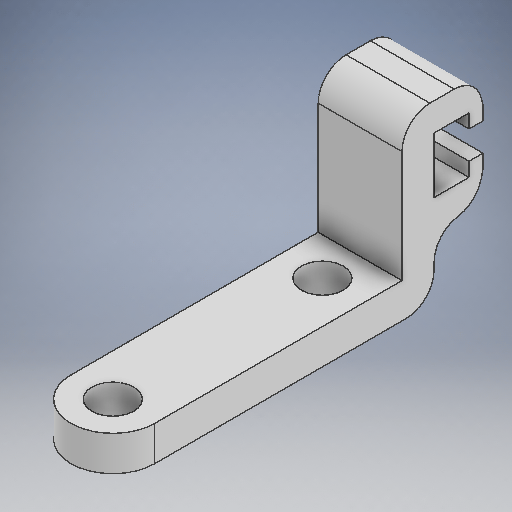
# Autodesk Inventor part: wire_holder_femur
Saved by Autodesk Inventor 2026.1 (Build 301233000, 233)
## iProperties
Created: 2025-12-05
Part Number: wire_holder_femur
Material: Generic
Document SubType Name: Modeling
Designer: emanuel
Density: 1 g/cm^3
Appearance: Default
Author: emanuel
Autodesk Inventor part; units mm, degrees
ref_plane "YZ Plane" through (0, 0, 0) normal (1, 0, 0) x (0, 1, 0)
ref_plane "XZ Plane" through (0, 0, 0) normal (0, 1, 0) x (-1, 0, 0)
ref_plane "XY Plane" through (0, 0, 0) normal (0, 0, 1) x (1, 0, 0)
sketch "Sketch1" plane through (0, 0, 0) normal (0, 1, 0) x (-1, 0, 0)
  circle A0 centre (0, 0) radius 1.5
  line L0 (0, 0) -> (0, -15)
  line L1 (0, 0) -> (15, 0) construction
  circle A1 centre (0, -15) radius 1.5
  line L2 (0, -15) -> (0, -17.5)
  line L3 (0, -17.5) -> (0, -20)
  circle A2 centre (0, 0) radius 3
  line L4 (3, 0) -> (-3, 0)
  line L5 (-3, 0) -> (-3, -20)
  line L6 (-3, -20) -> (3, -20)
  line L7 (3, -20) -> (3, 0)
  dimension "d6" = 6
  dimension "d0" = 3
  dimension "d1" = 15
  dimension "d2" = 90
  dimension "d3" = 3
  dimension "d4" = 2.5
  dimension "d5" = 2.5
  constraints: 16 end point, 3 coincident, 2 centre point, 2 horizontal, 2 parallel, 2 perpendicular, 2 point on line, 2 vertical, 3 other
  measures "d0" diameter of A0
  measures "d1" distance of L0.start L0.end
  measures "d2" angle of L0 L1
  measures "d3" diameter of A1
  measures "d4" distance of L2.start L2.end
  measures "d5" distance of L2.end L3.end
sketch "Sketch1 outline for Extrusion1" plane through (0, 0, 0) normal (0, 1, 0) x (-1, 0, 0)
  arc A0 (3, 0) -> (-3, 0) centre (0, 0) ccw
  line L0 (3, -20) -> (3, 0)
  line L1 (-3, 0) -> (-3, -20)
  line L2 (-3, -20) -> (3, -20)
  circle A1 centre (0, -15) radius 1.5
  circle A2 centre (0, 0) radius 1.5
extrude "Extrusion1" add sketch "Sketch1 outline for Extrusion1" along normal blind 2.5
sketch "Sketch2" plane through (0, 2.5, 0) normal (0, 1, 0) x (1, 0, 0)
  line L0 (3, 20) -> (-3, 20) projected
  line L1 (-3, 20) -> (3, 20)
  line L2 (3, 20) -> (3, 17.7)
  line L3 (3, 17.7) -> (-3, 17.7)
  line L4 (-3, 17.7) -> (-3, 20)
  point P0 (0, 0)
  dimension "d9" = 2.3
  constraints: 8 end point, 2 parallel, 1 horizontal, 1 perpendicular
  measures "d9" distance of L1.end L2.end
sketch "Sketch2 outline for Extrusion2" plane through (0, 2.5, 0) normal (0, 1, 0) x (1, 0, 0)
  line L0 (-3, 20) -> (-3, 17.7)
  line L1 (3, 20) -> (-3, 20)
  line L2 (3, 17.7) -> (3, 20)
  line L3 (-3, 17.7) -> (3, 17.7)
extrude "Extrusion2" add sketch "Sketch2 outline for Extrusion2" along normal blind 10
sketch "Sketch3" plane through (3, 0, -20) normal (0, 0, -1) x (-1, 0, 0)
  line L0 (0, 0) -> (0, 12.5) projected
  line L1 (6, 0) -> (6, 12.5) projected
  line L2 (0, 12.5) -> (6, 12.5)
  line L3 (6, 12.5) -> (6, 10.5)
  line L4 (6, 10.5) -> (0, 10.5)
  line L5 (0, 10.5) -> (0, 12.5)
  line L6 (0, 10.5) -> (6, 10.5)
  line L7 (6, 10.5) -> (6, 6.5)
  line L8 (6, 6.5) -> (0, 6.5)
  line L9 (0, 6.5) -> (0, 10.5)
  line L10 (0, 6.5) -> (6, 6.5)
  line L11 (6, 6.5) -> (6, 4.5)
  line L12 (6, 4.5) -> (0, 4.5)
  line L13 (0, 4.5) -> (0, 6.5)
  point P0 (3, 0)
  point P1 (0, 4.5)
  point P2 (0, 6.5)
  point P3 (0, 10.5)
  dimension "d12" = 2
  dimension "d13" = 6
  dimension "d14" = 4
  dimension "d15" = 2
  constraints: 24 end point, 6 parallel, 3 horizontal, 3 perpendicular, 2 point on line
  measures "d12" distance of L2.end L3.end
  measures "d13" distance of L7.end L8.end
  measures "d14" distance of L6.end L7.end
  measures "d15" distance of L10.end L11.end
sketch "Sketch3 outline for Extrusion3" plane through (3, 0, -20) normal (0, 0, -1) x (-1, 0, 0)
  line L0 (0, 4.5) -> (6, 4.5)
  line L1 (0, 6.5) -> (0, 4.5)
  line L2 (6, 6.5) -> (0, 6.5)
  line L3 (6, 4.5) -> (6, 6.5)
  line L4 (6, 12.5) -> (0, 12.5)
  line L5 (6, 10.5) -> (6, 12.5)
  line L6 (0, 10.5) -> (6, 10.5)
  line L7 (0, 12.5) -> (0, 10.5)
extrude "Extrusion3" add sketch "Sketch3 outline for Extrusion3" along normal blind 3
sketch "Sketch4" plane through (3, 0, 0) normal (1, 0, 0) x (0, 0, -1)
  line L0 (20, 10.5) -> (23, 10.5)
  line L1 (20, 6.5) -> (23, 6.5)
  line L2 (23, 10.5) -> (22.5, 10.5)
  line L3 (22.5, 10.5) -> (22.5, 6.5)
  line L4 (22.5, 6.5) -> (23, 6.5)
  line L5 (23, 6.5) -> (23, 10.5)
  line L6 (22.5, 10.5) -> (23.5, 10.5)
  line L7 (23.5, 10.5) -> (23.5, 9.5)
  line L8 (23.5, 9.5) -> (22.5, 9.5)
  line L9 (22.5, 9.5) -> (22.5, 10.5)
  line L10 (22.5, 6.5) -> (23.5, 6.5)
  line L11 (23.5, 6.5) -> (23.5, 7.5)
  line L12 (23.5, 7.5) -> (22.5, 7.5)
  line L13 (22.5, 7.5) -> (22.5, 6.5)
  line L14 (23, 12.5) -> (23, 10.5)
  line L15 (23.5, 10.5) -> (23, 12.5)
  line L16 (23, 12.5) -> (23, 10.5)
  line L17 (23.5, 6.5) -> (23, 4.499196)
  line L18 (23, 4.5) -> (23, 6.5)
  line L19 (23, 4.499196) -> (23, 6.5)
  point P0 (0, 0)
  dimension "d18" = 0.5
  dimension "d19" = 1
  dimension "d20" = 1
  dimension "d21" = 1
  dimension "d22" = 1
  constraints: 32 end point, 6 parallel, 3 horizontal, 3 perpendicular, 2 collinear, 1 point on line
  measures "d18" distance of L4.end L3.end
  measures "d19" distance of L7.end L8.end
  measures "d20" distance of L6.end L7.end
  measures "d21" distance of L12.end L11.end
  measures "d22" distance of L11.end L10.end
sketch "Sketch4 outline for Extrusion4" plane through (3, 0, 0) normal (1, 0, 0) x (0, 0, -1)
  line L0 (23, 4.5) -> (23.5, 6.5)
  line L1 (23, 6.5) -> (23, 4.5)
  line L2 (22.5, 6.5) -> (23, 6.5)
  line L3 (22.5, 7.5) -> (22.5, 6.5)
  line L4 (23.5, 7.5) -> (22.5, 7.5)
  line L5 (23.5, 6.5) -> (23.5, 7.5)
  line L6 (22.5, 9.5) -> (23.5, 9.5)
  line L7 (22.5, 10.5) -> (22.5, 9.5)
  line L8 (23, 10.5) -> (22.5, 10.5)
  line L9 (23, 12.5) -> (23, 10.5)
  line L10 (23.5, 10.5) -> (23, 12.5)
  line L11 (23.5, 9.5) -> (23.5, 10.5)
extrude "Extrusion4" add sketch "Sketch4 outline for Extrusion4" against normal blind 6
fillet "Fillet1" radius 2 5 edges at (0, 12.5, -23) (0, 12.5, -17.7) (0, 4.5, -23) (0, 4.5, -20) (0, 0, -20)
body "Solid1"
